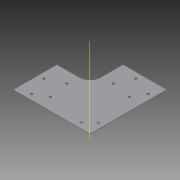
# Autodesk Inventor part: NickBracket
Saved by Autodesk Inventor 2015 (Build 190159000, 159)
## iProperties
Created: 2015-01-29
Part Number: NickBracket
Material: Generic
Document SubType Name: Modeling
Designer: pltwe4
Density: 1 g/cm^3
Appearance: Default
Author: pltwe4
Autodesk Inventor part; units mm, degrees
ref_plane "YZ Plane" through (0, 0, 0) normal (1, 0, 0) x (0, 1, 0)
ref_plane "XZ Plane" through (0, 0, 0) normal (0, 1, 0) x (-1, 0, 0)
ref_plane "XY Plane" through (0, 0, 0) normal (0, 0, 1) x (1, 0, 0)
sketch "Sketch1" plane through (0, 0, 0) normal (0, 1, 0) x (-1, 0, 0)
  line L0 (0, 0) -> (136.7536, 0)
  line L1 (136.7536, 0) -> (136.7536, -77.5208)
  line L2 (136.7536, -77.5208) -> (96.5708, -77.5208)
  line L3 (77.5208, -96.5708) -> (77.5208, -136.7536)
  line L4 (77.5208, -136.7536) -> (0, -136.7536)
  line L5 (0, -136.7536) -> (0, 0)
  arc A0 (96.5708, -77.5208) -> (77.5208, -96.5708) centre (96.5708, -96.5708) ccw
  circle A1 centre (9.525, -24.765) radius 2.2225
  circle A2 centre (24.765, -9.525) radius 2.2225
  circle A3 centre (9.525, -113.8936) radius 2.2225
  circle A4 centre (113.8936, -9.525) radius 2.2225
  circle A5 centre (126.5936, -44.45) radius 2.2225
  circle A6 centre (98.6536, -57.15) radius 2.2225
  circle A7 centre (92.3036, -21.59) radius 2.2225
  circle A8 centre (44.45, -126.5936) radius 2.2225
  circle A9 centre (57.15, -98.6536) radius 2.2225
  circle A10 centre (21.59, -92.3036) radius 2.2225
  line L6 (0, 0) -> (96.5708, -96.5708) construction
  dimension "d0" = 136.7536
  dimension "d1" = 77.5208
  dimension "d2" = 19.05
  dimension "d3" = 9.525
  dimension "d6" = 9.525
  dimension "d7" = 22.86
  dimension "d8" = 10.16
  dimension "d9" = 44.45
  dimension "d10" = 4.445
  dimension "d11" = 24.765
  dimension "d12" = 38.1
  dimension "d13" = 57.15
  dimension "d14" = 21.59
  dimension "d15" = 44.45
  constraints: 14 end point, 11 centre point, 8 equal radius, 7 perpendicular, 2 point on circle, 2 tangent, 1 horizontal, 5 other
  measures "d0" distance between parallel lines of L5 L1
  measures "d1" distance between parallel lines of L0 L2
  measures "d2" radius of A0
  measures "d3" distance from line of L5 A1.centre
  measures "d6" distance from line of L5 A3.centre
  measures "d7" distance from line of L4 A3.centre
  measures "d8" distance from line of L4 A8.centre
  measures "d9" distance from line of L5 A8.centre
  measures "d10" diameter of A1
  measures "d11" distance from line of L0 A1.centre
  measures "d12" distance from line of L4 A9.centre
  measures "d13" distance from line of L5 A9.centre
  measures "d14" distance from line of L5 A10.centre
  measures "d15" distance from line of L4 A10.centre
extrude "Extrusion1" add sketch "Sketch1" along normal blind 0.889
ref_plane "Work Plane1" through (0, 0, 0) normal (0.7071, 0, -0.7071) x (-0.7071, 0, -0.7071)
body "Solid1"
